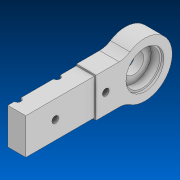
# Autodesk Inventor part: Bearing Holder Tracking Wheels
Saved by Autodesk Inventor 2022.2 (Build 262287000, 287)
## iProperties
Created: 2022-01-03
Part Number: Bearing Holder Tracking Wheels
Material: Generic
Document SubType Name: Modeling
Designer: omard
Density: 1 g/cm^3
Appearance: Default
Author: omard
Autodesk Inventor part; units mm, degrees
ref_plane "YZ Plane" through (0, 0, 0) normal (1, 0, 0) x (0, 1, 0)
ref_plane "XZ Plane" through (0, 0, 0) normal (0, 1, 0) x (-1, 0, 0)
ref_plane "XY Plane" through (0, 0, 0) normal (0, 0, 1) x (1, 0, 0)
sketch "Sketch1" plane through (0, 0, 0) normal (1, 0, 0) x (0, 1, 0)
  circle A0 centre (0, 0) radius 12.3063
  line L0 (11.684, 76.2) -> (-11.684, 76.2)
  line L1 (-11.684, 76.2) -> (-11.684, 31.75)
  line L2 (-11.684, 12.3063) -> (11.684, 12.3063) construction
  line L3 (11.684, 12.3063) -> (11.684, 13.2748) construction
  circle A1 centre (0, 0) radius 3.8354
  circle A2 centre (0, 0) radius 11.1125
  arc A3 (-11.684, 13.2748) -> (-12.7, 12.3063) centre (0, 0) ccw
  line L4 (12.7, 31.75) -> (-12.7, 31.75)
  line L5 (-12.7, 31.75) -> (-12.7, 12.3063)
  line L6 (-12.7, 12.3063) -> (12.7, 12.3063) construction
  line L7 (12.7, 12.3063) -> (12.7, 31.75)
  arc A4 (12.7, 16.6747) -> (14.7833, 9.705) centre (25.4, 16.6747) ccw
  arc A5 (-14.7833, 9.705) -> (-12.7, 16.6747) centre (-25.4, 16.6747) ccw
  arc A6 (11.684, 13.2748) -> (-11.684, 13.2748) centre (0, 0) ccw
  arc A7 (12.7, 12.3063) -> (11.684, 13.2748) centre (0, 0) ccw
  arc A8 (-12.7, 12.3063) -> (-14.7833, 9.705) centre (0, 0) ccw
  arc A9 (-14.7833, 9.705) -> (14.7833, 9.705) centre (0, 0) ccw
  arc A10 (14.7833, 9.705) -> (12.7, 12.3063) centre (0, 0) ccw
  line L8 (-11.684, 13.2748) -> (-11.684, 12.3063) construction
  line L9 (11.684, 13.2748) -> (11.684, 31.75) construction
  line L10 (-11.684, 31.75) -> (-11.684, 13.2748) construction
  line L11 (11.684, 31.75) -> (11.684, 76.2)
  circle A11 centre (0, 0) radius 6.35
  point P0 (0, 12.3063)
  point P1 (0, 12.3063)
  point P2 (-10.16, 25.0063)
  point P3 (11.684, 12.7)
  point P4 (10.16, 25.0063)
  dimension "d1" = 24.6126
  dimension "d2" = 7.6708
  dimension "d3" = 22.225
  dimension "d5" = 25.4
  dimension "d7" = 12.7
  dimension "d8" = 44.45
  dimension "d13" = 12.7
  dimension "d27" = 1.016
  dimension "d29" = 31.75
  constraints: 24 end point, 22 point on circle, 12 parallel, 11 centre point, 6 coincident, 4 perpendicular, 4 point on line, 4 tangent, 2 horizontal, 2 midpoint, 2 vertical alignment, 1 collinear, 1 equal radius, 2 other
  measures "d2" diameter of A1
  measures "d3" diameter of A2
  measures "d5" distance between parallel lines of L5 L7
  measures "d7" radius of A4
  measures "d8" distance between parallel lines of L0 L4
  measures "d13" diameter of A11
  measures "d27" distance between parallel lines of L7 L11
  measures "d29" distance from line of L4 point (0, 0)
extrude "Extrusion1" add sketch "Sketch1" along normal blind 11.684 contours L11 L4 L1 L0
extrude "Extrusion2" add sketch "Sketch1" along normal blind 12.7 contours L4 L7 A7 A6 A3 L5 | A4 A10 L7 | L5 A8 A5 | A10 A9 A8 A3 A6 A7
extrude "Extrusion3" add sketch "Sketch1" along normal blind 5.588 contours A2
extrude "Extrusion4" add sketch "Sketch1" along normal blind 11.1252 contours A0
sketch "Sketch2" plane through (12.7, 0, 0) normal (1, 0, 0) x (0, 0, -1)
  line L0 (-31.75, 12.7) -> (-31.75, -12.7) projected
  line L1 (-76.2, 11.684) -> (-76.2, -11.684) projected
  point P0 (0, 0)
  point P1 (-82.55, 0)
  point P2 (-57.15, 0)
  point P3 (-76.2, 0)
  point P4 (-25.4, 0)
  dimension "d19" = 25.4
  dimension "d37" = 25.4
  dimension "d39" = 31.75
  constraints: 3 horizontal alignment, 1 midpoint
  measures "d19" distance of point (-57.15, 0) point (-82.55, 0)
  measures "d37" distance from line of point (-57.15, 0) L0
  measures "d39" distance of point (-57.15, 0) point (-25.4, 0)
hole "Hole1" at (12.7, 0, 57.15) at (12.7, 0, 82.55) at (12.7, 0, 25.4) direction (-1, 0, 0) diameter 4.318 end through all start extended yes
sketch "Sketch3" plane through (0, 11.684, 76.2) normal (0, 1, 0) x (1, 0, 0)
  line L0 (0, 44.45) -> (0, 0) projected
  line L1 (0, 0) -> (11.684, 0) projected
  line L2 (0, 21.209) -> (11.684, 21.209) projected
  line L3 (0, 16.891) -> (11.684, 16.891) projected
  line L4 (11.684, 21.209) -> (11.684, 16.891) projected
  point P0 (0, 76.2)
  point P1 (0, 6.35)
  point P2 (11.684, 19.05)
  point P3 (0, 31.75)
  dimension "d38" = 12.7
  dimension "d40" = 25.4
  constraints: 2 point on line, 1 midpoint
  measures "d38" vertical distance of point (0, 6.35) point (11.684, 19.05)
  measures "d40" distance of point (0, 6.35) point (0, 31.75)
hole "Hole2" at (0, 11.684, 69.85) at (0, 11.684, 44.45) direction (0, -1, 0) diameter 4.318 end through all start extended yes
body "Solid1"
